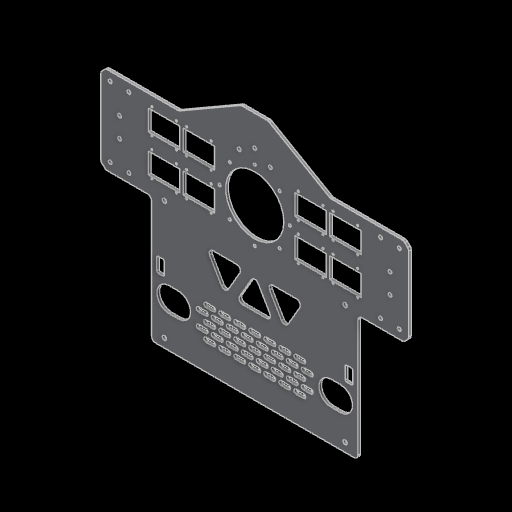
# Autodesk Inventor part: Root
Saved by Autodesk Inventor 2025.2 (Build 292293000, 293)
## iProperties
Created: 2020-05-07
Part Number: Root
Material: Generic
Document SubType Name: Sheet Metal
Designer: valer
Density: 1 g/cm^3
Sheet Metal Rule: Default
Appearance: Default
Author: valer
Autodesk Inventor part; units mm, degrees
ref_plane "YZ Plane" through (0, 0, 0) normal (1, 0, 0) x (0, 1, 0)
ref_plane "XZ Plane" through (0, 0, 0) normal (0, 1, 0) x (-1, 0, 0)
ref_plane "XY Plane" through (0, 0, 0) normal (0, 0, 1) x (1, 0, 0)
sketch "Base" plane through (0, 0, 0) normal (0, 0, 1) x (1, 0, 0)
  circle A0 centre (-56.25, 0) radius 2.75 construction
  circle A1 centre (0, -56.25) radius 2.75 construction
  circle A2 centre (0, 56.25) radius 2.75 construction
  circle A3 centre (39.7748, -39.7748) radius 2.75 construction
  circle A4 centre (-39.7748, 39.7748) radius 2.75 construction
  circle A5 centre (-39.7748, -39.7748) radius 2.75 construction
  circle A6 centre (39.7748, 39.7748) radius 2.75 construction
  circle A7 centre (56.25, 0) radius 2.75 construction
  circle A8 centre (0, 0) radius 45 construction
  circle A9 centre (0, 0) radius 61
  line L0 (0, -352) -> (0, 222) construction
  line L1 (-344.741, 0) -> (344.741, 0) construction
  circle A10 centre (0, 0) radius 46.5
  circle A11 centre (-56.25, 0) radius 2.25
  circle A12 centre (-39.7748, -39.7748) radius 2.25
  circle A13 centre (0, -56.25) radius 2.25
  circle A14 centre (39.7748, -39.7748) radius 2.25
  circle A15 centre (56.25, 0) radius 2.25
  circle A16 centre (39.7748, 39.7748) radius 2.25
  circle A17 centre (0, 56.25) radius 2.25
  circle A18 centre (-39.7748, 39.7748) radius 2.25
  line L2 (-121.2436, 70) -> (0, 140)
  line L3 (0, 140) -> (121.2436, 70)
  line L4 (121.2436, 70) -> (121.2436, -70)
  line L5 (121.2436, -70) -> (0, -140)
  line L6 (0, -140) -> (-121.2436, -70)
  line L7 (-121.2436, -70) -> (-121.2436, 70)
  line L8 (121.2436, 70) -> (246.2436, 70)
  line L9 (246.2436, 70) -> (246.2436, -70)
  line L10 (246.2436, -70) -> (121.2436, -70)
  line L11 (-121.2436, 70) -> (-246.2436, 70)
  line L12 (-246.2436, 70) -> (-246.2436, -70)
  line L13 (-246.2436, -70) -> (-121.2436, -70)
  line L14 (165, -70) -> (165, -270)
  line L15 (165, -270) -> (0, -270)
  line L16 (-165, -70) -> (-165, -270)
  line L17 (-165, -270) -> (0, -270)
  point P0 (0, 0)
  dimension "d91" = 1.5
  dimension "d92" = 4.5
  dimension "d164" = 125
  dimension "d165" = 140
  dimension "d173" = 165
  dimension "d174" = 200
  measures "d91" radial gap between concentric circles of A10 A8
  measures "d92" diameter of A11
  measures "d164" distance of L3.end L8.end
  measures "d165" distance of L8.end L9.end
  measures "d173" distance of L14.end L15.end
  measures "d174" distance between parallel lines of L10 L15
extrude "Plate1" add sketch "Base" against normal blind 4 contours A9 | L2 L3 L4 L5 L6 L7 | L7 L13 L12 L11 | L6 L5 L10 L14 L15 L17 L16 L13 | L8 L9 L10 L4
sketch "LegMountHoles" plane through (0, 0, -4) normal (0, 0, -1) x (-1, 0, 0)
  line L0 (-216.2436, 44.9096) -> (-216.2436, -35.0904) construction
  line L1 (-201.2436, 56) -> (-231.2436, 56) construction
  circle A0 centre (-201.2436, 56) radius 3
  circle A1 centre (-231.2436, 56) radius 3
  circle A2 centre (-216.2436, 16) radius 3
  line L2 (344.741, 0) -> (-344.741, 0) construction
  line L3 (0, -352) -> (0, 222) construction
  circle A3 centre (201.2436, 56) radius 3
  circle A4 centre (231.2436, 56) radius 3
  circle A5 centre (216.2436, 16) radius 3
  circle A6 centre (-201.2436, -56) radius 3
  circle A7 centre (-231.2436, -56) radius 3
  circle A8 centre (-216.2436, -16) radius 3
  circle A9 centre (201.2436, -56) radius 3
  circle A10 centre (231.2436, -56) radius 3
  circle A11 centre (216.2436, -16) radius 3
  line L4 (-246.2436, -70) -> (-246.2436, 70) projected
  point P0 (0, 0)
  point P1 (-216.2436, 56)
  dimension "d93" = 6
  dimension "d94" = 30
  dimension "d95" = 40
  dimension "d161" = 16
  dimension "d166" = 30
  constraints: 12 centre point, 9 symmetric about line, 4 end point, 2 coincident, 2 equal radius, 2 point on line, 1 horizontal, 1 midpoint, 1 perpendicular, 9 other
  measures "d93" diameter of A0
  measures "d94" distance of L1.start L1.end
  measures "d95" distance from line of L1 A2.centre
  measures "d161" distance from line of L2 A2.centre
  measures "d166" distance between parallel lines of L4 L0
extrude "LegMountHolesFeature" cut sketch "LegMountHoles" against normal blind 4
chamfer "FrontChamferFeature" distance 25 angle 45 1 edges at (0, 140, -2)
chamfer "SideChamfersFeature" distance 8 angle 45 4 edges at (246.2436, 70, -2) (246.2436, -70, -2) (-246.2436, 70, -2) (-246.2436, -70, -2)
fillet "FilletsFeature" radius 6 16 edges at (165, -270, -2) (-165, -270, -2) (-238.2436, -70, -2) (-246.2436, -62, -2) (-165, -70, -2) (165, -70, -2) (238.2436, -70, -2) (246.2436, -62, -2) (246.2436, 62, -2) (238.2436, 70, -2) (121.2436, 70, -2) (21.6506, 127.5, -2) (-21.6506, 127.5, -2) (-121.2436, 70, -2) (-238.2436, 70, -2) (-246.2436, 62, -2)
sketch "BatteryContactHoles" plane through (0, 0, -4) normal (0, 0, -1) x (-1, 0, 0)
  circle A0 centre (-129.1, -199.15) radius 18.4 construction
  circle A1 centre (129.1, -199.15) radius 18.4 construction
  circle A2 centre (129.1, -199.15) radius 19.4
  circle A3 centre (-129.1, -199.15) radius 19.4
  point P0 (0, 0)
  dimension "d199" = 1
  constraints: 2 centre point, 2 coincident, 1 equal radius
  measures "d199" radial gap between concentric circles of A2 A1
extrude "BatteryContactHolesFeature" cut sketch "BatteryContactHoles" against normal blind 4
sketch "BatteryStrapHoles" plane through (0, 0, -4) normal (0, 0, -1) x (-1, 0, 0)
  line L0 (-156.75, -148) -> (-144.75, -148)
  line L1 (-144.75, -148) -> (-144.75, -171.5)
  line L2 (-144.75, -171.5) -> (-156.75, -171.5)
  line L3 (-156.75, -171.5) -> (-156.75, -148)
  line L4 (0, -349.5) -> (0, 207) construction
  line L5 (-156.75, -148) -> (-152.25, -148) projected
  line L6 (-152.25, -171.5) -> (-156.75, -171.5) projected
  line L7 (156.75, -148) -> (144.75, -148)
  line L8 (144.75, -148) -> (144.75, -171.5)
  line L9 (144.75, -171.5) -> (156.75, -171.5)
  line L10 (156.75, -171.5) -> (156.75, -148)
  point P0 (0, 0)
  dimension "d204" = 12
  constraints: 16 end point, 4 symmetric about line, 2 parallel, 1 horizontal, 1 perpendicular
  measures "d204" distance of L0.start L0.end
extrude "BatteryStrapHolesFeature" cut sketch "BatteryStrapHoles" against normal blind 4
fillet "BatteryStrapHoleFilletsFeature" radius 2 8 edges at (156.75, -148, -2) (144.75, -148, -2) (156.75, -171.5, -2) (144.75, -171.5, -2) (-144.75, -148, -2) (-156.75, -148, -2) (-156.75, -171.5, -2) (-144.75, -171.5, -2)
sketch "BaseCuts" plane through (0, 0, -4) normal (0, 0, -1) x (-1, 0, 0)
  line L0 (-77.3649, -96.25) -> (-47.9201, -147.25)
  line L1 (-47.9201, -147.25) -> (-18.4752, -96.25)
  line L2 (-18.4752, -96.25) -> (-77.3649, -96.25)
  line L3 (-66.3953, -147.25) -> (-95.8401, -96.25)
  line L4 (-95.8401, -96.25) -> (-125.285, -147.25)
  line L5 (-125.285, -147.25) -> (-66.3953, -147.25)
  line L6 (0, -349.5) -> (0, 207) construction
  line L7 (77.3649, -96.25) -> (47.9201, -147.25)
  line L8 (47.9201, -147.25) -> (18.4752, -96.25)
  line L9 (18.4752, -96.25) -> (77.3649, -96.25)
  line L10 (66.3953, -147.25) -> (95.8401, -96.25)
  line L11 (95.8401, -96.25) -> (125.285, -147.25)
  line L12 (125.285, -147.25) -> (66.3953, -147.25)
  line L13 (359.0244, -147.25) -> (-330.4576, -147.25) construction
  line L14 (-125.285, -163.25) -> (-66.3953, -163.25)
  line L15 (-66.3953, -163.25) -> (-95.8401, -214.25)
  line L16 (-95.8401, -214.25) -> (-125.285, -163.25)
  line L17 (-66.3953, -147.25) -> (-66.3953, -163.25) construction
  line L18 (125.285, -163.25) -> (66.3953, -163.25)
  line L19 (66.3953, -163.25) -> (95.8401, -214.25)
  line L20 (95.8401, -214.25) -> (125.285, -163.25)
  line L21 (18.4752, -96.25) -> (-18.4752, -96.25) construction
  line L22 (0, -96.25) -> (29.4449, -147.25)
  line L23 (0, -96.25) -> (-29.4449, -147.25)
  line L24 (-29.4449, -147.25) -> (29.4449, -147.25)
  circle A0 centre (0, -56.25) radius 2.25 projected
  point P0 (0, 0)
  dimension "d218" = 60
  dimension "d219" = 60
  dimension "d242" = 51
  dimension "d244" = 16
  dimension "d246" = 16
  dimension "d247" = 60
  dimension "d248" = 60
  dimension "d255" = 16
  dimension "d256" = 40
  constraints: 46 end point, 9 symmetric about line, 7 horizontal, 3 equal length, 3 parallel, 1 midpoint, 1 vertical, 6 other
  measures "d218" angle of L5 L3
  measures "d219" angle of L4 L5
  measures "d242" distance from line of L5 L3.end
  measures "d244" distance between parallel lines of L3 L0
  measures "d246" distance between parallel lines of L14 L5
  measures "d247" angle of L15 L14
  measures "d248" angle of L16 L14
  measures "d255" distance between parallel lines of L22 L8
  measures "d256" distance from line of L21 A0.centre
extrude "BaseCutsFeature" cut sketch "BaseCuts" against normal blind 4 contours L2 L1 L0 | L7 L8 L9 | L22 L24 L23
fillet "BaseCutFilletsFeature" radius 6 9 edges at (18.4752, -96.25, -2) (77.3649, -96.25, -2) (47.9201, -147.25, -2) (-77.3649, -96.25, -2) (-18.4752, -96.25, -2) (-47.9201, -147.25, -2) (0, -96.25, -2) (-29.4449, -147.25, -2) (29.4449, -147.25, -2)
sketch "LaserMountHoles" plane through (0, 0, -4) normal (0, 0, -1) x (-1, 0, 0)
  circle A0 centre (25, 65) radius 3 projected
  circle A1 centre (0, 79) radius 3 projected
  circle A2 centre (-25, 65) radius 3 projected
  point P0 (0, 0)
extrude "LaserMountHolesFeature" cut sketch "LaserMountHoles" against normal blind 4
sketch "MotorDriverMountHoles" plane through (0, 0, -4) normal (0, 0, -1) x (-1, 0, 0)
  circle A0 centre (-164.6136, 14.0225) radius 1.65 projected
  circle A1 centre (-164.6136, 54.2225) radius 1.65 projected
  circle A2 centre (-125.2136, 14.0225) radius 1.65 projected
  circle A3 centre (-125.2136, 54.2225) radius 1.65 projected
  circle A4 centre (-125.2136, -5.2775) radius 1.65 projected
  circle A5 centre (-164.6136, -5.2775) radius 1.65 projected
  circle A6 centre (-164.6136, -45.4775) radius 1.65 projected
  circle A7 centre (-125.2136, -45.4775) radius 1.65 projected
  circle A8 centre (-109.1136, -45.4775) radius 1.65 projected
  circle A9 centre (-109.1136, -5.2775) radius 1.65 projected
  circle A10 centre (-69.7136, -5.2775) radius 1.65 projected
  circle A11 centre (-69.7136, -45.4775) radius 1.65 projected
  circle A12 centre (-109.1136, 14.0225) radius 1.65 projected
  circle A13 centre (-109.1136, 54.2225) radius 1.65 projected
  circle A14 centre (-69.7136, 54.2225) radius 1.65 projected
  circle A15 centre (-69.7136, 14.0225) radius 1.65 projected
  line L0 (0, -349.5) -> (0, 207) construction
  circle A16 centre (164.6136, 14.0225) radius 1.65
  circle A17 centre (164.6136, 54.2225) radius 1.65
  circle A18 centre (125.2136, 14.0225) radius 1.65
  circle A19 centre (125.2136, 54.2225) radius 1.65
  circle A20 centre (125.2136, -5.2775) radius 1.65
  circle A21 centre (164.6136, -5.2775) radius 1.65
  circle A22 centre (164.6136, -45.4775) radius 1.65
  circle A23 centre (125.2136, -45.4775) radius 1.65
  circle A24 centre (109.1136, -45.4775) radius 1.65
  circle A25 centre (109.1136, -5.2775) radius 1.65
  circle A26 centre (69.7136, -5.2775) radius 1.65
  circle A27 centre (69.7136, -45.4775) radius 1.65
  circle A28 centre (109.1136, 14.0225) radius 1.65
  circle A29 centre (109.1136, 54.2225) radius 1.65
  circle A30 centre (69.7136, 54.2225) radius 1.65
  circle A31 centre (69.7136, 14.0225) radius 1.65
  line L1 (-120.1636, 49.3725) -> (-169.6636, 49.3725) construction
  line L2 (-169.6636, 16.8725) -> (-120.1636, 16.8725) construction
  line L3 (-169.6636, 54.9725) -> (-169.6636, 13.0725) construction
  line L4 (-120.1636, 27.7325) -> (-120.1636, 54.9725) construction
  line L5 (-169.9136, 49.6225) -> (-119.9136, 49.6225)
  line L6 (-119.9136, 49.6225) -> (-119.9136, 16.6225)
  line L7 (-119.9136, 16.6225) -> (-169.9136, 16.6225)
  line L8 (-169.9136, 16.6225) -> (-169.9136, 49.6225)
  line L9 (-169.9136, 49.6225) -> (-119.9136, 16.6225) construction
  line L10 (-114.4136, 49.6225) -> (-64.4136, 49.6225)
  line L11 (-64.4136, 49.6225) -> (-64.4136, 16.6225)
  line L12 (-64.4136, 16.6225) -> (-114.4136, 16.6225)
  line L13 (-114.4136, 16.6225) -> (-114.4136, 49.6225)
  line L14 (-169.9136, -9.8775) -> (-119.9136, -9.8775)
  line L15 (-119.9136, -9.8775) -> (-119.9136, -42.8775)
  line L16 (-119.9136, -42.8775) -> (-169.9136, -42.8775)
  line L17 (-169.9136, -42.8775) -> (-169.9136, -9.8775)
  line L18 (-114.4136, -9.8775) -> (-64.4136, -9.8775)
  line L19 (-64.4136, -9.8775) -> (-64.4136, -42.8775)
  line L20 (-64.4136, -42.8775) -> (-114.4136, -42.8775)
  line L21 (-114.4136, -42.8775) -> (-114.4136, -9.8775)
  line L22 (169.9136, 49.6225) -> (119.9136, 49.6225)
  line L23 (119.9136, 49.6225) -> (119.9136, 16.6225)
  line L24 (119.9136, 16.6225) -> (169.9136, 16.6225)
  line L25 (169.9136, 16.6225) -> (169.9136, 49.6225)
  line L26 (114.4136, 49.6225) -> (64.4136, 49.6225)
  line L27 (64.4136, 49.6225) -> (64.4136, 16.6225)
  line L28 (64.4136, 16.6225) -> (114.4136, 16.6225)
  line L29 (114.4136, 16.6225) -> (114.4136, 49.6225)
  line L30 (169.9136, -9.8775) -> (119.9136, -9.8775)
  line L31 (119.9136, -9.8775) -> (119.9136, -42.8775)
  line L32 (119.9136, -42.8775) -> (169.9136, -42.8775)
  line L33 (169.9136, -42.8775) -> (169.9136, -9.8775)
  line L34 (114.4136, -9.8775) -> (64.4136, -9.8775)
  line L35 (64.4136, -9.8775) -> (64.4136, -42.8775)
  line L36 (64.4136, -42.8775) -> (114.4136, -42.8775)
  line L37 (114.4136, -42.8775) -> (114.4136, -9.8775)
  point P0 (0, 0)
  dimension "d259" = 0.25
  dimension "d260" = 0.25
  dimension "d261" = 0.25
  dimension "d262" = 0.25
  dimension "d263" = 50
  dimension "d264" = 33
  dimension "d265" = 2.6
  dimension "d266" = 5.3
  dimension "d267" = 5.3
  dimension "d268" = 5.3
  dimension "d269" = 5.3
  dimension "d270" = 2.6
  constraints: 66 end point, 32 symmetric about line, 16 centre point, 8 parallel, 6 equal length, 4 horizontal, 4 perpendicular, 2 point on line, 1 collinear, 16 other
  measures "d259" distance between parallel lines of L7 L2
  measures "d260" distance between parallel lines of L8 L3
  measures "d261" distance between parallel lines of L5 L1
  measures "d262" distance between parallel lines of L6 L4
  measures "d263" distance of L6.end L7.end
  measures "d264" distance of L7.end L5.start
  measures "d265" distance from line of L7 A2.centre
  measures "d266" distance from line of A2.centre L6
  measures "d267" distance from line of L11 A15.centre
  measures "d268" distance from line of A7.centre L15
  measures "d269" distance from line of L19 A11.centre
  measures "d270" distance from line of A7.centre L16
extrude "MotorDriverHolesFeature" cut sketch "MotorDriverMountHoles" against normal blind 4
sketch "VentHoles" plane through (0, 0, -4) normal (0, 0, -1) x (-1, 0, 0)
  line L0 (344.741, 0) -> (-344.741, 0) construction
  line L1 (0, -349.5) -> (0, 207) construction
  line L2 (-6, -177.0913) -> (6, -177.0913) construction
  line L3 (-6, -180.5913) -> (6, -180.5913)
  line L4 (6, -173.5913) -> (-6, -173.5913)
  arc A0 (-6, -173.5913) -> (-6, -180.5913) centre (-6, -177.0913) ccw
  arc A1 (6, -180.5913) -> (6, -173.5913) centre (6, -177.0913) ccw
  arc A2 (-30, -173.5913) -> (-30, -180.5913) centre (-30, -177.0913) ccw
  line L5 (-18, -173.5913) -> (-30, -173.5913)
  line L6 (-30, -180.5913) -> (-18, -180.5913)
  arc A3 (-18, -180.5913) -> (-18, -173.5913) centre (-18, -177.0913) ccw
  arc A4 (18, -173.5913) -> (18, -180.5913) centre (18, -177.0913) ccw
  line L7 (30, -173.5913) -> (18, -173.5913)
  line L8 (18, -180.5913) -> (30, -180.5913)
  arc A5 (30, -180.5913) -> (30, -173.5913) centre (30, -177.0913) ccw
  arc A6 (-54, -173.5913) -> (-54, -180.5913) centre (-54, -177.0913) ccw
  line L9 (-42, -173.5913) -> (-54, -173.5913)
  line L10 (-54, -180.5913) -> (-42, -180.5913)
  arc A7 (-42, -180.5913) -> (-42, -173.5913) centre (-42, -177.0913) ccw
  arc A8 (42, -173.5913) -> (42, -180.5913) centre (42, -177.0913) ccw
  line L11 (54, -173.5913) -> (42, -173.5913)
  line L12 (42, -180.5913) -> (54, -180.5913)
  arc A9 (54, -180.5913) -> (54, -173.5913) centre (54, -177.0913) ccw
  arc A10 (-78, -173.5913) -> (-78, -180.5913) centre (-78, -177.0913) ccw
  line L13 (-66, -173.5913) -> (-78, -173.5913)
  line L14 (-78, -180.5913) -> (-66, -180.5913)
  arc A11 (-66, -180.5913) -> (-66, -173.5913) centre (-66, -177.0913) ccw
  arc A12 (66, -173.5913) -> (66, -180.5913) centre (66, -177.0913) ccw
  line L15 (78, -173.5913) -> (66, -173.5913)
  line L16 (66, -180.5913) -> (78, -180.5913)
  arc A13 (78, -180.5913) -> (78, -173.5913) centre (78, -177.0913) ccw
  line L17 (0, -189.0913) -> (-165, -189.0913) construction
  line L18 (-165, -264) -> (-165, -76) projected
  line L19 (-6, -197.5913) -> (6, -197.5913)
  line L20 (6, -204.5913) -> (-6, -204.5913)
  arc A14 (-6, -197.5913) -> (-6, -204.5913) centre (-6, -201.0913) ccw
  arc A15 (6, -204.5913) -> (6, -197.5913) centre (6, -201.0913) ccw
  arc A16 (-30, -197.5913) -> (-30, -204.5913) centre (-30, -201.0913) ccw
  line L21 (-18, -204.5913) -> (-30, -204.5913)
  line L22 (-30, -197.5913) -> (-18, -197.5913)
  arc A17 (-18, -204.5913) -> (-18, -197.5913) centre (-18, -201.0913) ccw
  arc A18 (18, -197.5913) -> (18, -204.5913) centre (18, -201.0913) ccw
  line L23 (30, -204.5913) -> (18, -204.5913)
  line L24 (18, -197.5913) -> (30, -197.5913)
  arc A19 (30, -204.5913) -> (30, -197.5913) centre (30, -201.0913) ccw
  arc A20 (-54, -197.5913) -> (-54, -204.5913) centre (-54, -201.0913) ccw
  line L25 (-42, -204.5913) -> (-54, -204.5913)
  line L26 (-54, -197.5913) -> (-42, -197.5913)
  arc A21 (-42, -204.5913) -> (-42, -197.5913) centre (-42, -201.0913) ccw
  arc A22 (42, -197.5913) -> (42, -204.5913) centre (42, -201.0913) ccw
  line L27 (54, -204.5913) -> (42, -204.5913)
  line L28 (42, -197.5913) -> (54, -197.5913)
  arc A23 (54, -204.5913) -> (54, -197.5913) centre (54, -201.0913) ccw
  arc A24 (-78, -197.5913) -> (-78, -204.5913) centre (-78, -201.0913) ccw
  line L29 (-66, -204.5913) -> (-78, -204.5913)
  line L30 (-78, -197.5913) -> (-66, -197.5913)
  arc A25 (-66, -204.5913) -> (-66, -197.5913) centre (-66, -201.0913) ccw
  arc A26 (66, -197.5913) -> (66, -204.5913) centre (66, -201.0913) ccw
  line L31 (78, -204.5913) -> (66, -204.5913)
  line L32 (66, -197.5913) -> (78, -197.5913)
  arc A27 (78, -204.5913) -> (78, -197.5913) centre (78, -201.0913) ccw
  line L33 (-6, -201.0913) -> (6, -201.0913) construction
  line L34 (-6, -221.5913) -> (6, -221.5913)
  line L35 (6, -228.5913) -> (-6, -228.5913)
  arc A28 (-6, -221.5913) -> (-6, -228.5913) centre (-6, -225.0913) ccw
  arc A29 (6, -228.5913) -> (6, -221.5913) centre (6, -225.0913) ccw
  arc A30 (-30, -221.5913) -> (-30, -228.5913) centre (-30, -225.0913) ccw
  line L36 (-18, -228.5913) -> (-30, -228.5913)
  line L37 (-30, -221.5913) -> (-18, -221.5913)
  arc A31 (-18, -228.5913) -> (-18, -221.5913) centre (-18, -225.0913) ccw
  arc A32 (18, -221.5913) -> (18, -228.5913) centre (18, -225.0913) ccw
  line L38 (30, -228.5913) -> (18, -228.5913)
  line L39 (18, -221.5913) -> (30, -221.5913)
  arc A33 (30, -228.5913) -> (30, -221.5913) centre (30, -225.0913) ccw
  arc A34 (-54, -221.5913) -> (-54, -228.5913) centre (-54, -225.0913) ccw
  line L40 (-42, -228.5913) -> (-54, -228.5913)
  line L41 (-54, -221.5913) -> (-42, -221.5913)
  arc A35 (-42, -228.5913) -> (-42, -221.5913) centre (-42, -225.0913) ccw
  arc A36 (42, -221.5913) -> (42, -228.5913) centre (42, -225.0913) ccw
  line L42 (54, -228.5913) -> (42, -228.5913)
  line L43 (42, -221.5913) -> (54, -221.5913)
  arc A37 (54, -228.5913) -> (54, -221.5913) centre (54, -225.0913) ccw
  arc A38 (-78, -221.5913) -> (-78, -228.5913) centre (-78, -225.0913) ccw
  line L44 (-66, -228.5913) -> (-78, -228.5913)
  line L45 (-78, -221.5913) -> (-66, -221.5913)
  arc A39 (-66, -228.5913) -> (-66, -221.5913) centre (-66, -225.0913) ccw
  arc A40 (66, -221.5913) -> (66, -228.5913) centre (66, -225.0913) ccw
  line L46 (78, -228.5913) -> (66, -228.5913)
  line L47 (66, -221.5913) -> (78, -221.5913)
  arc A41 (78, -228.5913) -> (78, -221.5913) centre (78, -225.0913) ccw
  line L48 (-18, -189.0913) -> (-6, -189.0913) construction
  line L49 (-18, -192.5913) -> (-6, -192.5913)
  line L50 (-6, -185.5913) -> (-18, -185.5913)
  arc A42 (-18, -185.5913) -> (-18, -192.5913) centre (-18, -189.0913) ccw
  arc A43 (-6, -192.5913) -> (-6, -185.5913) centre (-6, -189.0913) ccw
  line L51 (-30, -185.5913) -> (-42, -185.5913)
  arc A44 (-30, -192.5913) -> (-30, -185.5913) centre (-30, -189.0913) ccw
  line L52 (-42, -192.5913) -> (-30, -192.5913)
  arc A45 (-42, -185.5913) -> (-42, -192.5913) centre (-42, -189.0913) ccw
  line L53 (-54, -185.5913) -> (-66, -185.5913)
  arc A46 (-54, -192.5913) -> (-54, -185.5913) centre (-54, -189.0913) ccw
  line L54 (-66, -192.5913) -> (-54, -192.5913)
  arc A47 (-66, -185.5913) -> (-66, -192.5913) centre (-66, -189.0913) ccw
  line L55 (-78, -185.5913) -> (-90, -185.5913)
  arc A48 (-78, -192.5913) -> (-78, -185.5913) centre (-78, -189.0913) ccw
  line L56 (-90, -192.5913) -> (-78, -192.5913)
  arc A49 (-90, -185.5913) -> (-90, -192.5913) centre (-90, -189.0913) ccw
  line L57 (18, -192.5913) -> (6, -192.5913)
  line L58 (6, -185.5913) -> (18, -185.5913)
  arc A50 (18, -192.5913) -> (18, -185.5913) centre (18, -189.0913) ccw
  arc A51 (6, -185.5913) -> (6, -192.5913) centre (6, -189.0913) ccw
  line L59 (30, -185.5913) -> (42, -185.5913)
  arc A52 (30, -185.5913) -> (30, -192.5913) centre (30, -189.0913) ccw
  line L60 (42, -192.5913) -> (30, -192.5913)
  arc A53 (42, -192.5913) -> (42, -185.5913) centre (42, -189.0913) ccw
  line L61 (54, -185.5913) -> (66, -185.5913)
  arc A54 (54, -185.5913) -> (54, -192.5913) centre (54, -189.0913) ccw
  line L62 (66, -192.5913) -> (54, -192.5913)
  arc A55 (66, -192.5913) -> (66, -185.5913) centre (66, -189.0913) ccw
  line L63 (78, -185.5913) -> (90, -185.5913)
  arc A56 (78, -185.5913) -> (78, -192.5913) centre (78, -189.0913) ccw
  line L64 (90, -192.5913) -> (78, -192.5913)
  arc A57 (90, -192.5913) -> (90, -185.5913) centre (90, -189.0913) ccw
  line L65 (-18, -209.5913) -> (-6, -209.5913)
  line L66 (-6, -216.5913) -> (-18, -216.5913)
  arc A58 (-18, -209.5913) -> (-18, -216.5913) centre (-18, -213.0913) ccw
  arc A59 (-6, -216.5913) -> (-6, -209.5913) centre (-6, -213.0913) ccw
  line L67 (-30, -216.5913) -> (-42, -216.5913)
  arc A60 (-30, -216.5913) -> (-30, -209.5913) centre (-30, -213.0913) ccw
  line L68 (-42, -209.5913) -> (-30, -209.5913)
  arc A61 (-42, -209.5913) -> (-42, -216.5913) centre (-42, -213.0913) ccw
  line L69 (-54, -216.5913) -> (-66, -216.5913)
  arc A62 (-54, -216.5913) -> (-54, -209.5913) centre (-54, -213.0913) ccw
  line L70 (-66, -209.5913) -> (-54, -209.5913)
  arc A63 (-66, -209.5913) -> (-66, -216.5913) centre (-66, -213.0913) ccw
  line L71 (-78, -216.5913) -> (-90, -216.5913)
  arc A64 (-78, -216.5913) -> (-78, -209.5913) centre (-78, -213.0913) ccw
  line L72 (-90, -209.5913) -> (-78, -209.5913)
  arc A65 (-90, -209.5913) -> (-90, -216.5913) centre (-90, -213.0913) ccw
  line L73 (78, -216.5913) -> (90, -216.5913)
  arc A66 (90, -216.5913) -> (90, -209.5913) centre (90, -213.0913) ccw
  line L74 (90, -209.5913) -> (78, -209.5913)
  arc A67 (78, -209.5913) -> (78, -216.5913) centre (78, -213.0913) ccw
  arc A68 (66, -216.5913) -> (66, -209.5913) centre (66, -213.0913) ccw
  line L75 (54, -216.5913) -> (66, -216.5913)
  line L76 (66, -209.5913) -> (54, -209.5913)
  arc A69 (54, -209.5913) -> (54, -216.5913) centre (54, -213.0913) ccw
  arc A70 (42, -216.5913) -> (42, -209.5913) centre (42, -213.0913) ccw
  line L77 (30, -216.5913) -> (42, -216.5913)
  line L78 (42, -209.5913) -> (30, -209.5913)
  arc A71 (30, -209.5913) -> (30, -216.5913) centre (30, -213.0913) ccw
  arc A72 (18, -216.5913) -> (18, -209.5913) centre (18, -213.0913) ccw
  line L79 (18, -209.5913) -> (6, -209.5913)
  line L80 (6, -216.5913) -> (18, -216.5913)
  arc A73 (6, -209.5913) -> (6, -216.5913) centre (6, -213.0913) ccw
  point P0 (0, 0)
  point P1 (0, -177.0913)
  point P2 (-12, -189.0913)
  dimension "d271" = 3.5
  dimension "d272" = 177.0913
  dimension "d273" = 12
  dimension "d276" = 24
  dimension "d281" = 12
  dimension "d282" = 12
  dimension "d285" = 24
  constraints: 160 end point, 156 symmetric about line, 148 point on circle, 74 centre point, 8 tangent, 5 point on line, 4 horizontal, 3 parallel, 2 midpoint, 1 equal radius, 1 perpendicular, 142 other
  measures "d271" radius of A1
  measures "d272" distance between parallel lines of L2 L0
  measures "d273" distance of L4.start L4.end
  measures "d276" distance of L2.start A2.centre
  measures "d281" distance between parallel lines of L17 L2
  measures "d282" distance from line of L1 point (-12, -189.091)
  measures "d285" distance of L50.start L51.start
extrude "VentHolesFeature" cut sketch "VentHoles" against normal blind 4
sketch "BatteryContactsExtend" plane through (0, 0, -4) normal (0, 0, -1) x (-1, 0, 0)
  circle A0 centre (-129.1, -199.15) radius 19.4 projected
  circle A1 centre (129.1, -199.15) radius 19.4 projected
  line L0 (-129.1, -199.15) -> (129.1, -199.15) construction
  line L1 (-137, -199.15) -> (-122, -199.15) construction
  line L2 (-137, -218.5459) -> (-122, -218.5459)
  line L3 (-122, -179.7541) -> (-137, -179.7541)
  arc A2 (-137, -179.7541) -> (-137, -218.5459) centre (-137, -199.15) ccw
  arc A3 (-122, -218.5459) -> (-122, -179.7541) centre (-122, -199.15) ccw
  line L4 (-165, -264) -> (-165, -76) projected
  line L5 (0, -349.5) -> (0, 207) construction
  line L6 (137, -218.5459) -> (122, -218.5459)
  line L7 (122, -179.7541) -> (137, -179.7541)
  arc A4 (137, -218.5459) -> (137, -179.7541) centre (137, -199.15) ccw
  arc A5 (122, -179.7541) -> (122, -218.5459) centre (122, -199.15) ccw
  point P0 (0, 0)
  point P1 (-129.5, -199.15)
  point P2 (-129.5, -179.7541)
  dimension "d292" = 28
  dimension "d293" = 15
  constraints: 14 end point, 8 point on circle, 6 symmetric about line, 4 centre point, 4 tangent, 2 midpoint, 2 parallel, 1 horizontal, 1 point on line, 4 other
  measures "d292" distance from line of L4 L1.start
  measures "d293" distance of L1.start L1.end
extrude "BatteryContactsExtendFeature" cut sketch "BatteryContactsExtend" against normal blind 4 contours A0 L2 L3 | A0 L3 A3 L2 | A0 L2 A2 L3 | A1 L6 L7 | A1 L7 A4 L6 | A1 L6 A5 L7
sketch "BatteryMountHoles" plane through (0, 0, -4) normal (0, 0, -1) x (-1, 0, 0)
  ellipse E0 centre (-144.491, -256) end of major axis (-144.491, -259.5) minor radius 3.5 projected
  ellipse E1 centre (144.509, -256) end of major axis (144.509, -259.5) minor radius 3.5 projected
  ellipse E2 centre (-144.491, -66) end of major axis (-144.491, -69.5) minor radius 3.5 projected
  ellipse E3 centre (144.509, -66) end of major axis (144.509, -69.5) minor radius 3.5 projected
  point P0 (0, 0)
extrude "BatteryMountHolesFeature" cut sketch "BatteryMountHoles" against normal blind 4
equation "\"d97\" = Thickness"
equation "\"d33\" = Thickness"
equation "\"BendRadius\" = Thickness"
equation "\"BendReliefWidth\" = Thickness"
equation "\"BendReliefDepth\" = 0.5 * Thickness"
equation "\"CornerReliefSize\" = 4 * Thickness"
equation "\"MinimumRemnant\" = 2 * Thickness"
equation "\"TransitionRadius\" = BendRadius"
equation "\"JacobiRadiusSize\" = BendRadius"
equation "\"GapSize\" = Thickness"
equation "\"Thickness\" = 4"
body "Solid1"
